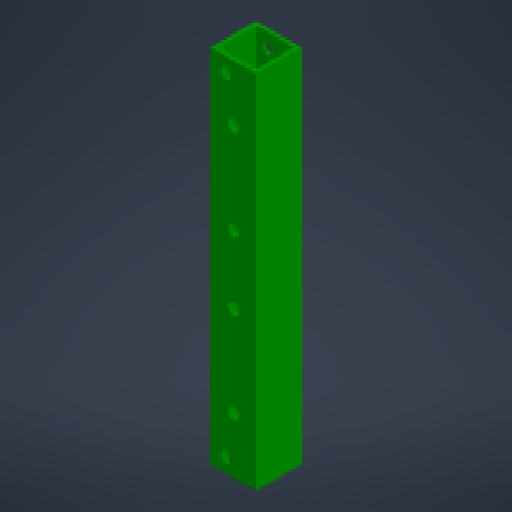
# Autodesk Inventor part: main axis
Saved by Autodesk Inventor 2024 (Build 280153000, 153)
## iProperties
Created: 2023-04-17
Part Number: main axis
Material: Типовые
Document SubType Name: Modeling
Designer: user
Density: 1 g/cm^3
Appearance: По умолчанию
Author: user
Autodesk Inventor part; units mm, degrees
ref_plane "YZ Plane" through (0, 0, 0) normal (1, 0, 0) x (0, 1, 0)
ref_plane "XZ Plane" through (0, 0, 0) normal (0, 1, 0) x (-1, 0, 0)
ref_plane "XY Plane" through (0, 0, 0) normal (0, 0, 1) x (1, 0, 0)
sketch "Эскиз1" plane through (0, 0, 0) normal (0, 0, 1) x (1, 0, 0)
  line L0 (0, 0) -> (-20, 0)
  line L1 (-20, 0) -> (-20, 20)
  line L2 (-20, 20) -> (0, 20)
  line L3 (0, 20) -> (0, 0)
  line L4 (-1.5, 1.5) -> (-18.5, 1.5)
  line L5 (-18.5, 1.5) -> (-18.5, 18.5)
  line L6 (-18.5, 18.5) -> (-1.5, 18.5)
  line L7 (-1.5, 18.5) -> (-1.5, 1.5)
  point P0 (-10, 18.5)
  point P1 (-10, 20)
  point P2 (-18.5, 10)
  point P3 (-20, 10)
  dimension "d0" = 20
  dimension "d1" = 1.5
  constraints: 16 end point, 4 midpoint, 4 parallel, 4 perpendicular, 2 horizontal, 1 horizontal alignment, 1 vertical alignment
  measures "d0" distance of L1.end L2.end
  measures "d1" horizontal distance of L1.end L5.end
extrude "Выдавливание3" add sketch "Эскиз1" against normal blind 160
sketch "Эскиз3" plane through (-20, 0, 0) normal (0, -1, 0) x (1, 0, 0)
  circle A0 centre (10, -25) radius 2.5 projected
  circle A1 centre (10, -65) radius 2.5 projected
  circle A2 centre (10, -95) radius 2.5 projected
  circle A3 centre (10, -135) radius 2.5 projected
  point P0 (20, 0)
extrude "Выдавливание4" cut sketch "Эскиз3" against normal through all
sketch "Эскиз4" plane through (-20, 20, 0) normal (0, 1, 0) x (1, 0, 0)
  circle A0 centre (6.5, 153.5) radius 2.25
  circle A1 centre (6.5, 6.5) radius 2.25
  point P0 (20, 0)
  constraints: 2 centre point, 4 other
extrude "Выдавливание5" cut sketch "Эскиз4" against normal through all
